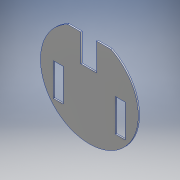
# Autodesk Inventor part: Cuerpo
Saved by Autodesk Inventor 2016 (Build 200138000, 138)
## iProperties
Created: 2019-03-15
Part Number: Cuerpo
Material: Aluminio 6061
Document SubType Name: Modeling
Designer: FIMCP
Mass: 79.9853 g
Surface Area: 312.511 cm^2
Volume: 29.6242 cm^3
Density: 2.7 g/cm^3
Appearance: Aluminio - Plano
Author: FIMCP
Autodesk Inventor part; units mm, degrees
ref_plane "YZ Plane" through (0, 0, 0) normal (1, 0, 0) x (0, 1, 0)
ref_plane "XZ Plane" through (0, 0, 0) normal (0, 1, 0) x (-1, 0, 0)
ref_plane "XY Plane" through (0, 0, 0) normal (0, 0, 1) x (1, 0, 0)
sketch "Boceto1" plane through (0, 0, 0) normal (0, 1, 0) x (-1, 0, 0)
  arc A0 (-18, 72.808) -> (20, 72.2842) centre (0, 0) ccw
  line L0 (-18, 72.808) -> (-18, 72.2842)
  line L1 (-11, 25) -> (13, 25)
  line L2 (55, 8) -> (40, 8)
  line L3 (40, 8) -> (40, -42)
  line L4 (40, -42) -> (55, -42)
  line L5 (55, -42) -> (55, 8)
  line L6 (-40, 8) -> (-55, 8)
  line L7 (-55, 8) -> (-55, -42)
  line L8 (-55, -42) -> (-40, -42)
  line L9 (-40, -42) -> (-40, 8)
  line L10 (20, 72.2842) -> (13, 72.2842)
  line L11 (13, 72.2842) -> (13, 25)
  line L12 (-18, 72.808) -> (-11, 72.808)
  line L13 (-11, 72.808) -> (-11, 25)
  line L14 (-18, 72.2842) -> (-18, 72.808)
  dimension "d0" = 150
  dimension "d2" = 18
  dimension "d3" = 25
  dimension "d4" = 15
  dimension "d5" = 50
  dimension "d6" = 15
  dimension "d7" = 50
  dimension "d8" = 40
  dimension "d9" = 40
  dimension "d63" = 8
  dimension "d64" = 8
  constraints: 30 end point, 5 parallel, 4 horizontal, 4 perpendicular, 2 point on circle, 1 centre point, 1 coincident, 1 point on line
  measures "d0" diameter of A0
  measures "d2" distance from line of L0 point (0, 0)
  measures "d3" distance from line of L1 point (0, 0)
  measures "d4" distance of L4.end L3.end
  measures "d5" distance of L3.end L2.end
  measures "d6" distance of L8.end L7.end
  measures "d7" distance of L7.end L6.end
  measures "d8" distance from line of L9 point (0, 0)
  measures "d9" distance from line of L3 point (0, 0)
  measures "d63" distance from line of point (0, 0) L2
  measures "d64" distance from line of point (0, 0) L6
extrude "Extrusión1" add sketch "Boceto1" along normal blind 2
sketch "Boceto8" plane through (0, 0, 0) normal (0, 1, 0) x (-1, 0, 0)
  line L0 (59.5508, 67.2842) -> (-59.748, 67.2842)
  line L1 (-59.748, 67.2842) -> (-59.748, 82.2842)
  line L2 (-59.748, 82.2842) -> (59.5508, 82.2842)
  line L3 (59.5508, 82.2842) -> (59.5508, 67.2842)
  line L4 (13, 72.2842) -> (20, 72.2842) projected
  point P0 (0, 0)
  dimension "d67" = 15
  dimension "d71" = 5
  constraints: 8 end point, 2 parallel, 1 horizontal, 1 perpendicular
  measures "d67" distance of L0.end L1.end
  measures "d71" distance between parallel lines of L4 L0
extrude "Extrusión8" cut sketch "Boceto8" along normal mid plane 70
